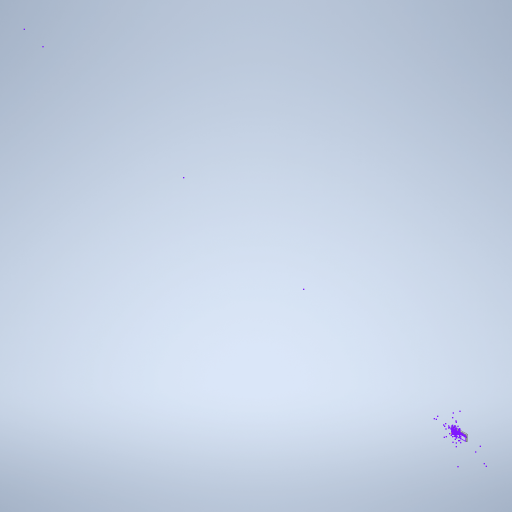
# Autodesk Inventor part: stump
Saved by Autodesk Inventor 2024 (Build 280153000, 153)
## iProperties
Created: 2023-12-16
Part Number: stump
Material: 一般
Document SubType Name: Modeling
Designer: right
Density: 1 g/cm^3
Appearance: 既定
Author: right
Autodesk Inventor part; units mm, degrees
(part 1 of 5)
ref_plane "YZ Plane" through (0, 0, 0) normal (1, 0, 0) x (0, 1, 0)
ref_plane "XZ Plane" through (0, 0, 0) normal (0, 1, 0) x (-1, 0, 0)
ref_plane "XY Plane" through (0, 0, 0) normal (0, 0, 1) x (1, 0, 0)
sketch "スケッチ1" plane through (0, 0, 0) normal (0, 0, 1) x (1, 0, 0)
  line L0 (2, 26.7042) -> (70.8408, 26.7042) construction
  line L1 (70.8408, 26.7042) -> (70.8408, 2) construction
  line L2 (70.8408, 2) -> (2, 2) construction
  line L3 (2, 2) -> (2, 26.7042) construction
  line L4 (0, 28.7042) -> (72.8408, 28.7042)
  line L5 (72.8408, 28.7042) -> (72.8408, 0)
  line L6 (72.8408, 0) -> (0, 0)
  line L7 (0, 0) -> (0, 28.7042)
  point P0 (36.4204, 28.7042)
  point P1 (0, 14.3521)
  point P2 (72.8408, 14.3521)
  dimension "d0" = 2
  dimension "d1" = 2
  dimension "d2" = 2
  dimension "d3" = 2
  dimension "d4" = 24.7042
  dimension "d5" = 68.8408
  constraints: 8 end point, 3 midpoint, 2 parallel, 1 coincident, 1 horizontal, 1 perpendicular, 2 other
  measures "d0" distance between parallel lines of L4 L0
  measures "d1" distance between parallel lines of L3 L7
  measures "d2" distance between parallel lines of L5 L1
  measures "d3" distance between parallel lines of L2 L6
  measures "d4" distance of L2.end L0.start
  measures "d5" distance of L0.start L0.end
extrude "押し出し1" add sketch "スケッチ1" along normal blind 5
sketch "スケッチ3" plane through (0, 0, 5) normal (0, 0, 1) x (1, 0, 0)
  line L0 (4.2953, 20.9134) -> (4.2763, 20.7484)
  line L1 (4.2763, 20.7484) -> (3.4513, 20.7317)
  line L2 (3.4513, 20.7317) -> (2.6263, 20.715)
  line L3 (2.6263, 20.715) -> (2.6263, 20.4784)
  line L4 (2.6263, 20.4784) -> (2.6263, 20.2418)
  line L5 (2.6263, 20.2418) -> (3.4464, 20.2251)
  arc A0 (3.8346, 20.2134) -> (3.4464, 20.2251) centre (3.0385, 0.191) ccw
  arc A1 (4.0836, 20.195) -> (3.8346, 20.2134) centre (3.6895, 16.5634) ccw
  arc A2 (4.2485, 20.1707) -> (4.0836, 20.195) centre (3.8458, 18.004) ccw
  arc A3 (4.2914, 20.1334) -> (4.2485, 20.1707) centre (4.2383, 20.1158) ccw
  arc A4 (4.2735, 20.0969) -> (4.2914, 20.1334) centre (4.2638, 20.1243) ccw
  arc A5 (4.1799, 20.0746) -> (4.2735, 20.0969) centre (4.121, 20.5302) ccw
  arc A6 (4.0094, 20.0617) -> (4.1799, 20.0746) centre (3.9733, 21.6725) ccw
  arc A7 (3.7113, 20.0584) -> (4.0094, 20.0617) centre (3.7113, 33.3375) ccw
  line L6 (3.7113, 20.0584) -> (3.1063, 20.0584)
  line L7 (3.1063, 20.0584) -> (3.1063, 19.2184)
  line L8 (3.1063, 19.2184) -> (3.1063, 18.3784)
  line L9 (3.1063, 18.3784) -> (3.4513, 18.3759)
  line L10 (3.4513, 18.3759) -> (3.7963, 18.3735)
  line L11 (3.7963, 18.3735) -> (3.5375, 18.1395)
  arc A8 (3.418, 18.0423) -> (3.5375, 18.1395) centre (2.5532, 19.2279) ccw
  arc A9 (3.2722, 17.9436) -> (3.418, 18.0423) centre (1.9502, 20.0545) ccw
  arc A10 (3.1239, 17.8579) -> (3.2722, 17.9436) centre (1.9972, 19.9794) ccw
  arc A11 (2.9975, 17.8013) -> (3.1239, 17.8579) centre (2.6369, 18.7749) ccw
  arc A12 (2.9975, 17.8013) -> (2.8882, 17.7602) centre (7.4649, 5.7405) ccw
  arc A13 (2.8882, 17.7602) -> (2.7926, 17.7231) centre (5.6156, 10.5973) ccw
  arc A14 (2.7926, 17.7231) -> (2.7116, 17.6907) centre (7.9302, 4.755) ccw
  arc A15 (2.7116, 17.6907) -> (2.6949, 17.6814) centre (2.7402, 17.6199) ccw
  arc A16 (2.6949, 17.6814) -> (2.6919, 17.6673) centre (2.7013, 17.6727) ccw
  arc A17 (2.6919, 17.6673) -> (2.7367, 17.5912) centre (5.8636, 19.479) ccw
  arc A18 (2.7367, 17.5912) -> (2.7944, 17.5007) centre (4.586, 18.7076) ccw
  arc A19 (2.7944, 17.5007) -> (2.8671, 17.3963) centre (6.3161, 19.8732) ccw
  arc A20 (2.8671, 17.3963) -> (2.9831, 17.2428) centre (6.0578, 19.6877) ccw
  arc A21 (2.9831, 17.2428) -> (3.053, 17.1803) centre (3.2002, 17.4155) ccw
  arc A22 (3.053, 17.1803) -> (3.1199, 17.1636) centre (3.1123, 17.2751) ccw
  arc A23 (3.1199, 17.1636) -> (3.208, 17.1828) centre (3.0992, 17.469) ccw
  arc A24 (3.208, 17.1828) -> (3.3895, 17.2713) centre (2.8086, 18.2332) ccw
  arc A25 (3.3895, 17.2713) -> (3.6464, 17.4363) centre (0.5309, 22.0048) ccw
  arc A26 (3.6464, 17.4363) -> (3.907, 17.6251) centre (0.4768, 22.0841) ccw
  arc A27 (3.907, 17.6251) -> (4.1113, 17.7989) centre (2.2399, 19.7922) ccw
  line L12 (4.1113, 17.7989) -> (4.3063, 17.9819)
  line L13 (4.3063, 17.9819) -> (4.3063, 17.5502)
  line L14 (4.3063, 17.5502) -> (4.3063, 17.1184)
  line L15 (4.3063, 17.1184) -> (4.6063, 17.1184)
  line L16 (4.6063, 17.1184) -> (4.9063, 17.1184)
  line L17 (4.9063, 17.1184) -> (4.9063, 17.5398)
  line L18 (4.9063, 17.5398) -> (4.9063, 17.9612)
  line L19 (4.9063, 17.9612) -> (5.1947, 17.7332)
  arc A28 (5.1947, 17.7332) -> (5.3299, 17.633) centre (6.8616, 19.842) ccw
  arc A29 (5.3299, 17.633) -> (5.4996, 17.5198) centre (8.6049, 22.3563) ccw
  arc A30 (5.4996, 17.5198) -> (5.6748, 17.4117) centre (8.642, 22.4141) ccw
  arc A31 (5.6748, 17.4117) -> (5.8276, 17.3268) centre (7.2249, 20.025) ccw
  line L20 (5.8276, 17.3268) -> (6.1722, 17.1484)
  line L21 (6.1722, 17.1484) -> (6.3476, 17.3584)
  arc A32 (6.3476, 17.3584) -> (6.4148, 17.4432) centre (4.7299, 18.7098) ccw
  arc A33 (6.4148, 17.4432) -> (6.4717, 17.5243) centre (5.2305, 18.3335) ccw
  arc A34 (6.4717, 17.5243) -> (6.5143, 17.594) centre (5.2832, 18.2992) ccw
  arc A35 (6.5143, 17.594) -> (6.5236, 17.6284) centre (6.4531, 17.6291) ccw
  arc A36 (6.5236, 17.6284) -> (6.5083, 17.6587) centre (6.4867, 17.6288) ccw
  arc A37 (6.5083, 17.6587) -> (6.4283, 17.7122) centre (5.7202, 16.5665) ccw
  arc A38 (6.4283, 17.7122) -> (6.3231, 17.7711) centre (5.6981, 16.5306) ccw
  arc A39 (6.3231, 17.7711) -> (6.1982, 17.8295) centre (5.257, 15.6552) ccw
  arc A40 (6.0567, 17.8982) -> (6.1982, 17.8295) centre (6.9163, 19.4888) ccw
  arc A41 (5.9009, 17.9884) -> (6.0567, 17.8982) centre (7.526, 20.6168) ccw
  arc A42 (5.7548, 18.0847) -> (5.9009, 17.9884) centre (7.4687, 20.5241) ccw
  arc A43 (5.6442, 18.172) -> (5.7548, 18.0847) centre (6.4837, 19.1222) ccw
  line L22 (5.6442, 18.172) -> (5.4163, 18.3734)
  line L23 (5.4163, 18.3734) -> (5.7613, 18.3759)
  line L24 (5.7613, 18.3759) -> (6.1063, 18.3784)
  line L25 (6.1063, 18.3784) -> (6.1063, 19.2184)
  line L26 (6.1063, 19.2184) -> (6.1063, 20.0584)
  line L27 (6.1063, 20.0584) -> (5.5063, 20.0584)
  arc A44 (5.1853, 20.0617) -> (5.5063, 20.0584) centre (5.5063, 35.6031) ccw
  arc A45 (5.0213, 20.0756) -> (5.1853, 20.0617) centre (5.2118, 21.3458) ccw
  arc A46 (4.935, 20.1024) -> (5.0213, 20.0756) centre (5.0654, 20.3701) ccw
  arc A47 (4.9063, 20.1484) -> (4.935, 20.1024) centre (4.9574, 20.1484) ccw
  arc A48 (4.9404, 20.196) -> (4.9063, 20.1484) centre (4.9565, 20.1484) ccw
  arc A49 (5.0563, 20.2217) -> (4.9404, 20.196) centre (5.1171, 19.6747) ccw
  arc A50 (5.2734, 20.2353) -> (5.0563, 20.2217) centre (5.3051, 17.9825) ccw
  arc A51 (5.7163, 20.2384) -> (5.2734, 20.2353) centre (5.7162, -11.2951) ccw
  line L28 (5.7163, 20.2384) -> (6.5263, 20.2384)
  line L29 (6.5263, 20.2384) -> (6.5263, 20.4784)
  line L30 (6.5263, 20.4784) -> (6.5263, 20.7184)
  line L31 (6.5263, 20.7184) -> (5.7163, 20.7184)
  line L32 (5.7163, 20.7184) -> (4.9063, 20.7184)
  line L33 (4.9063, 20.7184) -> (4.9063, 20.8984)
  arc A52 (4.9063, 20.8984) -> (4.8979, 21.0074) centre (4.1924, 20.8984) ccw
  arc A53 (4.8979, 21.0074) -> (4.8666, 21.0543) centre (4.8319, 20.9972) ccw
  arc A54 (4.8666, 21.0543) -> (4.7992, 21.0746) centre (4.7936, 20.9342) ccw
  arc A55 (4.7992, 21.0746) -> (4.6103, 21.0784) centre (4.6103, 16.3512) ccw
  arc A56 (4.6103, 21.0784) -> (4.4295, 21.0742) centre (4.6103, 17.1725) ccw
  arc A57 (4.4295, 21.0742) -> (4.3551, 21.0541) centre (4.4377, 20.8964) ccw
  arc A58 (4.3551, 21.0541) -> (4.3163, 21.0085) centre (4.3922, 20.9832) ccw
  arc A59 (4.3163, 21.0085) -> (4.2953, 20.9134) centre (4.7646, 20.8594) ccw
  arc A60 (4.2646, 19.4728) -> (4.2913, 19.5034) centre (4.2414, 19.52) ccw
  arc A61 (4.2012, 19.4492) -> (4.2646, 19.4728) centre (4.115, 19.7769) ccw
  arc A62 (4.1132, 19.4335) -> (4.2012, 19.4492) centre (4.0607, 19.983) ccw
  arc A63 (4.0063, 19.4284) -> (4.1132, 19.4335) centre (4.0063, 20.5531) ccw
  arc A64 (3.8994, 19.4335) -> (4.0063, 19.4284) centre (4.0063, 20.5531) ccw
  arc A65 (3.8114, 19.4492) -> (3.8994, 19.4335) centre (3.9518, 19.983) ccw
  arc A66 (3.7479, 19.4728) -> (3.8114, 19.4492) centre (3.8976, 19.7769) ccw
  arc A67 (3.7213, 19.5034) -> (3.7479, 19.4728) centre (3.7712, 19.52) ccw
  arc A68 (3.7302, 19.5372) -> (3.7213, 19.5034) centre (3.7516, 19.5135) ccw
  arc A69 (3.7741, 19.561) -> (3.7302, 19.5372) centre (3.8009, 19.4589) ccw
  arc A70 (3.8618, 19.5746) -> (3.7741, 19.561) centre (3.8842, 19.1424) ccw
  arc A71 (4.0063, 19.5784) -> (3.8618, 19.5746) centre (4.0063, 16.7936) ccw
  arc A72 (4.1508, 19.5746) -> (4.0063, 19.5784) centre (4.0063, 16.7936) ccw
  arc A73 (4.2385, 19.561) -> (4.1508, 19.5746) centre (4.1283, 19.1424) ccw
  arc A74 (4.2824, 19.5372) -> (4.2385, 19.561) centre (4.2116, 19.4589) ccw
  arc A75 (4.2913, 19.5034) -> (4.2824, 19.5372) centre (4.261, 19.5135) ccw
  arc A76 (5.4647, 19.4729) -> (5.4916, 19.5034) centre (5.4425, 19.5196) ccw
  arc A77 (5.3927, 19.4449) -> (5.4647, 19.4729) centre (5.2397, 19.945) ccw
  arc A78 (5.2969, 19.4226) -> (5.3927, 19.4449) centre (5.182, 20.1337) ccw
  arc A79 (5.1866, 19.4101) -> (5.2969, 19.4226) centre (5.1106, 20.5756) ccw
  arc A80 (5.0427, 19.4046) -> (5.1866, 19.4101) centre (5.012, 22.0861) ccw
  arc A81 (4.9634, 19.4146) -> (5.0427, 19.4046) centre (5.0394, 19.6984) ccw
  arc A82 (4.9222, 19.441) -> (4.9634, 19.4146) centre (4.9842, 19.4924) ccw
  arc A83 (4.9063, 19.4851) -> (4.9222, 19.441) centre (4.9754, 19.4851) ccw
  arc A84 (4.9238, 19.5297) -> (4.9063, 19.4851) centre (4.9718, 19.4851) ccw
  arc A85 (4.9703, 19.5588) -> (4.9238, 19.5297) centre (5.0013, 19.4576) ccw
  arc A86 (5.0579, 19.5743) -> (4.9703, 19.5588) centre (5.0775, 19.2085) ccw
  arc A87 (5.2113, 19.5784) -> (5.0579, 19.5743) centre (5.2113, 16.7018) ccw
  arc A88 (5.3531, 19.5746) -> (5.2113, 19.5784) centre (5.2113, 16.9114) ccw
  arc A89 (5.4395, 19.5609) -> (5.3531, 19.5746) centre (5.3307, 19.1545) ccw
  arc A90 (5.4828, 19.5371) -> (5.4395, 19.5609) centre (5.4127, 19.4608) ccw
  arc A91 (5.4916, 19.5034) -> (5.4828, 19.5371) centre (5.4611, 19.5134) ccw
  arc A92 (4.2894, 18.955) -> (4.3063, 18.9784) centre (4.2816, 18.9784) ccw
  arc A93 (4.2182, 18.936) -> (4.2894, 18.955) centre (4.103, 19.5117) ccw
  arc A94 (4.1213, 18.9227) -> (4.2182, 18.936) centre (4.061, 19.722) ccw
  arc A95 (4.0063, 18.9184) -> (4.1213, 18.9227) centre (4.0063, 20.4468) ccw
  arc A96 (3.8913, 18.9227) -> (4.0063, 18.9184) centre (4.0063, 20.4468) ccw
  arc A97 (3.7944, 18.936) -> (3.8913, 18.9227) centre (3.9516, 19.722) ccw
  arc A98 (3.7231, 18.955) -> (3.7944, 18.936) centre (3.9095, 19.5117) ccw
  arc A99 (3.7063, 18.9784) -> (3.7231, 18.955) centre (3.7309, 18.9784) ccw
  arc A100 (3.7231, 19.0018) -> (3.7063, 18.9784) centre (3.7309, 18.9784) ccw
  arc A101 (3.7944, 19.0208) -> (3.7231, 19.0018) centre (3.9095, 18.4451) ccw
  arc A102 (3.8913, 19.0341) -> (3.7944, 19.0208) centre (3.9516, 18.2348) ccw
  arc A103 (4.0063, 19.0384) -> (3.8913, 19.0341) centre (4.0063, 17.51) ccw
  arc A104 (4.1213, 19.0341) -> (4.0063, 19.0384) centre (4.0063, 17.51) ccw
  arc A105 (4.2182, 19.0208) -> (4.1213, 19.0341) centre (4.061, 18.2348) ccw
  arc A106 (4.2894, 19.0018) -> (4.2182, 19.0208) centre (4.103, 18.4451) ccw
  arc A107 (4.3063, 18.9784) -> (4.2894, 19.0018) centre (4.2816, 18.9784) ccw
  arc A108 (5.4894, 18.955) -> (5.5063, 18.9784) centre (5.4816, 18.9784) ccw
  arc A109 (5.4182, 18.936) -> (5.4894, 18.955) centre (5.303, 19.5117) ccw
  arc A110 (5.3213, 18.9227) -> (5.4182, 18.936) centre (5.261, 19.722) ccw
  arc A111 (5.2063, 18.9184) -> (5.3213, 18.9227) centre (5.2063, 20.4468) ccw
  arc A112 (5.0913, 18.9227) -> (5.2063, 18.9184) centre (5.2063, 20.4468) ccw
  arc A113 (4.9944, 18.936) -> (5.0913, 18.9227) centre (5.1516, 19.722) ccw
  arc A114 (4.9231, 18.955) -> (4.9944, 18.936) centre (5.1095, 19.5117) ccw
  arc A115 (4.9063, 18.9784) -> (4.9231, 18.955) centre (4.9309, 18.9784) ccw
  arc A116 (4.9231, 19.0018) -> (4.9063, 18.9784) centre (4.9309, 18.9784) ccw
  arc A117 (4.9944, 19.0208) -> (4.9231, 19.0018) centre (5.1095, 18.4451) ccw
  arc A118 (5.0913, 19.0341) -> (4.9944, 19.0208) centre (5.1516, 18.2348) ccw
  arc A119 (5.2063, 19.0384) -> (5.0913, 19.0341) centre (5.2063, 17.51) ccw
  arc A120 (5.3213, 19.0341) -> (5.2063, 19.0384) centre (5.2063, 17.51) ccw
  arc A121 (5.4182, 19.0208) -> (5.3213, 19.0341) centre (5.261, 18.2348) ccw
  arc A122 (5.4894, 19.0018) -> (5.4182, 19.0208) centre (5.303, 18.4451) ccw
  arc A123 (5.5063, 18.9784) -> (5.4894, 19.0018) centre (5.4816, 18.9784) ccw
  line L34 (8.6863, 20.8684) -> (8.6863, 20.6584)
  line L35 (8.6863, 20.6584) -> (7.8463, 20.6584)
  line L36 (7.8463, 20.6584) -> (7.0063, 20.6584)
  line L37 (7.0063, 20.6584) -> (7.0063, 20.3884)
  line L38 (7.0063, 20.3884) -> (7.0063, 20.1184)
  line L39 (7.0063, 20.1184) -> (8.9563, 20.1184)
  line L40 (8.9563, 20.1184) -> (10.9063, 20.1184)
  line L41 (10.9063, 20.1184) -> (10.9063, 20.3884)
  line L42 (10.9063, 20.3884) -> (10.9063, 20.6584)
  line L43 (10.9063, 20.6584) -> (10.0963, 20.6584)
  line L44 (10.0963, 20.6584) -> (9.2863, 20.6584)
  line L45 (9.2863, 20.6584) -> (9.2863, 20.8684)
  line L46 (9.2863, 20.8684) -> (9.2863, 21.0784)
  line L47 (9.2863, 21.0784) -> (8.9863, 21.0784)
  line L48 (8.9863, 21.0784) -> (8.6863, 21.0784)
  line L49 (8.6863, 21.0784) -> (8.6863, 20.8684)
  line L50 (12.1063, 20.8384) -> (12.1063, 20.5984)
  line L51 (12.1063, 20.5984) -> (11.8063, 20.5984)
  line L52 (11.8063, 20.5984) -> (11.5063, 20.5984)
  line L53 (11.5063, 20.5984) -> (11.5063, 20.3284)
  line L54 (11.5063, 20.3284) -> (11.5063, 20.0584)
  line L55 (11.5063, 20.0584) -> (11.8063, 20.0584)
  arc A124 (11.9213, 20.0541) -> (11.8063, 20.0584) centre (11.8063, 18.53) ccw
  arc A125 (12.0182, 20.0408) -> (11.9213, 20.0541) centre (11.861, 19.2548) ccw
  arc A126 (12.0894, 20.0218) -> (12.0182, 20.0408) centre (11.903, 19.4651) ccw
  arc A127 (12.1063, 19.9984) -> (12.0894, 20.0218) centre (12.0816, 19.9984) ccw
  arc A128 (12.0881, 19.9747) -> (12.1063, 19.9984) centre (12.0817, 19.9984) ccw
  arc A129 (12.0013, 19.9559) -> (12.0881, 19.9747) centre (11.8495, 20.8665) ccw
  arc A130 (11.8853, 19.9427) -> (12.0013, 19.9559) centre (11.8157, 21.0694) ccw
  arc A131 (11.7463, 19.9384) -> (11.8853, 19.9427) centre (11.7463, 22.1938) ccw
  line L56 (11.7463, 19.9384) -> (11.3863, 19.9384)
  line L57 (11.3863, 19.9384) -> (11.3863, 19.6684)
  line L58 (11.3863, 19.6684) -> (11.3863, 19.3984)
  line L59 (11.3863, 19.3984) -> (11.8167, 19.3984)
  line L60 (11.8167, 19.3984) -> (12.2472, 19.3984)
  line L61 (12.2472, 19.3984) -> (12.1159, 19.2586)
  arc A132 (12.0459, 19.1953) -> (12.1159, 19.2586) centre (11.6911, 19.6577) ccw
  arc A133 (11.9396, 19.1189) -> (12.0459, 19.1953) centre (10.7798, 20.8453) ccw
  arc A134 (11.8188, 19.0431) -> (11.9396, 19.1189) centre (10.6517, 21.0359) ccw
  arc A135 (11.7004, 18.9795) -> (11.8188, 19.0431) centre (10.8993, 20.6131) ccw
  arc A136 (11.7004, 18.9795) -> (11.5902, 18.9251) centre (22.1341, -2.2983) ccw
  arc A137 (11.5902, 18.9251) -> (11.4945, 18.8771) centre (17.6879, 6.6513) ccw
  arc A138 (11.4945, 18.8771) -> (11.4126, 18.8354) centre (25.1822, -8.1426) ccw
  arc A139 (11.4126, 18.8354) -> (11.3986, 18.8266) centre (11.4539, 18.7545) ccw
  arc A140 (11.3986, 18.8266) -> (11.3934, 18.8135) centre (11.4069, 18.8157) ccw
  arc A141 (11.3934, 18.8135) -> (11.4069, 18.7341) centre (15.6569, 19.5007) ccw
  arc A142 (11.4069, 18.7341) -> (11.426, 18.64) centre (13.6642, 19.1413) ccw
  arc A143 (11.426, 18.64) -> (11.4519, 18.5309) centre (15.5791, 19.5701) ccw
  arc A144 (11.4519, 18.5309) -> (11.4937, 18.3833) centre (13.9854, 19.1688) ccw
  arc A145 (11.4937, 18.3833) -> (11.5309, 18.3093) centre (11.7412, 18.4613) ccw
  arc A146 (11.5309, 18.3093) -> (11.5753, 18.2784) centre (11.5972, 18.3573) ccw
  arc A147 (11.5753, 18.2784) -> (11.6346, 18.278) centre (11.6058, 18.3882) ccw
  arc A148 (11.6941, 18.2678) -> (11.6346, 18.278) centre (11.6532, 18.2071) ccw
  arc A149 (11.7291, 18.2158) -> (11.6941, 18.2678) centre (11.6475, 18.1988) ccw
  arc A150 (11.7436, 18.0852) -> (11.7291, 18.2158) centre (11.0515, 18.0744) ccw
  arc A151 (11.7463, 17.7428) -> (11.7436, 18.0852) centre (-10.0958, 17.7428) ccw
  line L62 (11.7463, 17.7428) -> (11.7463, 17.1784)
  line L63 (11.7463, 17.1784) -> (12.0463, 17.1784)
  arc A152 (12.0463, 17.1784) -> (12.2148, 17.1823) centre (12.0463, 20.8261) ccw
  arc A153 (12.2148, 17.1823) -> (12.2938, 17.1994) centre (12.2036, 17.4248) ccw
  arc A154 (12.2938, 17.1994) -> (12.3322, 17.2356) centre (12.267, 17.2664) ccw
  arc A155 (12.3322, 17.2356) -> (12.3463, 17.2984) centre (12.1989, 17.2984) ccw
  arc A156 (12.3683, 17.3633) -> (12.3463, 17.2984) centre (12.4527, 17.2984) ccw
  arc A157 (12.425, 17.3999) -> (12.3683, 17.3633) centre (12.4481, 17.302) ccw
  arc A158 (12.5482, 17.4154) -> (12.425, 17.3999) centre (12.5597, 16.8274) ccw
  arc A159 (12.8563, 17.4184) -> (12.5482, 17.4154) centre (12.8563, 1.6492) ccw
  line L64 (12.8563, 17.4184) -> (13.3663, 17.4184)
  line L65 (13.3663, 17.4184) -> (13.3663, 18.2884)
  line L66 (13.3663, 18.2884) -> (13.3663, 19.1584)
  line L67 (13.3663, 19.1584) -> (13.087, 19.1584)
  arc A160 (12.9007, 19.1601) -> (13.087, 19.1584) centre (13.087, 29.2397) ccw
  arc A161 (12.8581, 19.174) -> (12.9007, 19.1601) centre (12.9021, 19.2365) ccw
  arc A162 (12.8536, 19.2022) -> (12.8581, 19.174) centre (12.8696, 19.1903) ccw
  arc A163 (12.9163, 19.2784) -> (12.8536, 19.2022) centre (13.6915, 18.5768) ccw
  arc A164 (12.9789, 19.3313) -> (12.9163, 19.2784) centre (13.1448, 19.0716) ccw
  arc A165 (13.0561, 19.3688) -> (12.9789, 19.3313) centre (13.178, 19.0196) ccw
  arc A166 (13.1494, 19.3911) -> (13.0561, 19.3688) centre (13.2117, 18.9231) ccw
  arc A167 (13.26, 19.3984) -> (13.1494, 19.3911) centre (13.26, 18.5599) ccw
  line L68 (13.26, 19.3984) -> (13.4952, 19.3984)
  line L69 (13.4952, 19.3984) -> (13.4792, 19.6989)
  arc A168 (13.478, 19.8229) -> (13.4792, 19.6989) centre (14.9277, 19.7758) ccw
  arc A169 (13.4881, 19.9345) -> (13.478, 19.8229) centre (14.446, 19.7914) ccw
  arc A170 (13.5071, 20.0236) -> (13.4881, 19.9345) centre (14.2099, 19.8267) ccw
  arc A171 (13.5348, 20.0709) -> (13.5071, 20.0236) centre (13.6112, 19.9945) ccw
  arc A172 (13.5721, 20.0577) -> (13.5348, 20.0709) centre (13.5503, 20.0554) ccw
  arc A173 (13.5913, 19.8102) -> (13.5721, 20.0577) centre (9.1456, 19.5895) ccw
  arc A174 (13.6033, 19.3928) -> (13.5913, 19.8102) centre (3.594, 19.314) ccw
  arc A175 (13.6063, 18.6304) -> (13.6033, 19.3928) centre (-83.1975, 18.6304) ccw
  line L70 (13.6063, 18.6304) -> (13.6063, 17.1184)
  line L71 (13.6063, 17.1184) -> (13.9063, 17.1184)
  line L72 (13.9063, 17.1184) -> (14.2063, 17.1184)
  line L73 (14.2063, 17.1184) -> (14.2063, 18.7084)
  line L74 (14.2063, 18.7084) -> (14.2063, 20.2984)
  line L75 (14.2063, 20.2984) -> (14.4434, 20.2984)
  line L76 (14.4434, 20.2984) -> (14.6805, 20.2984)
  line L77 (14.6805, 20.2984) -> (14.593, 20.0134)
  arc A176 (14.5546, 19.8882) -> (14.593, 20.0134) centre (-1289.7906, 420.4583) ccw
  arc A177 (14.5113, 19.7473) -> (14.5546, 19.8882) centre (-2056.7606, 655.9978) ccw
  arc A178 (14.4699, 19.6126) -> (14.5113, 19.7473) centre (-1967.312, 628.522) ccw
  arc A179 (14.4378, 19.5079) -> (14.4699, 19.6126) centre (-712.7507, 243.0535) ccw
  arc A180 (14.4378, 19.5079) -> (14.4081, 19.3727) centre (15.244, 19.26) ccw
  arc A181 (14.4081, 19.3727) -> (14.4088, 19.2573) centre (14.8181, 19.3174) ccw
  arc A182 (14.4088, 19.2573) -> (14.4428, 19.1194) centre (15.1413, 19.3649) ccw
  arc A183 (14.4428, 19.1194) -> (14.5281, 18.8922) centre (19.778, 20.9939) ccw
  arc A184 (14.6638, 18.5071) -> (14.5281, 18.8922) centre (10.0238, 17.089) ccw
  arc A185 (14.6749, 18.2941) -> (14.6638, 18.5071) centre (14.2424, 18.3783) ccw
  arc A186 (14.5827, 18.1798) -> (14.6749, 18.2941) centre (14.5207, 18.3241) ccw
  arc A187 (14.3814, 18.1384) -> (14.5827, 18.1798) centre (14.3814, 18.6487) ccw
  arc A188 (14.3814, 18.1384) -> (14.3039, 18.126) centre (14.3814, 17.8911) ccw
  arc A189 (14.3039, 18.126) -> (14.2749, 18.0893) centre (14.3173, 18.0856) ccw
  arc A190 (14.2749, 18.0893) -> (14.2823, 18.0105) centre (14.4947, 18.0701) ccw
  arc A191 (14.2823, 18.0105) -> (14.35, 17.7784) centre (25.3033, 21.1009) ccw
  arc A192 (14.35, 17.7784) -> (14.4059, 17.613) centre (17.0017, 18.5827) ccw
  arc A193 (14.4059, 17.613) -> (14.4515, 17.5474) centre (14.5573, 17.6696) ccw
  arc A194 (14.4515, 17.5474) -> (14.5184, 17.5192) centre (14.5283, 17.6361) ccw
  arc A195 (14.5184, 17.5192) -> (14.6535, 17.5156) centre (14.616, 18.6659) ccw
  arc A196 (14.6535, 17.5156) -> (14.9602, 17.5767) centre (14.6223, 18.4729) ccw
  arc A197 (14.9602, 17.5767) -> (15.1627, 17.7314) centre (14.8039, 17.9913) ccw
  arc A198 (15.1627, 17.7314) -> (15.265, 17.9912) centre (14.7089, 18.0601) ccw
  arc A199 (15.265, 17.9912) -> (15.2712, 18.3686) centre (13.5086, 18.2088) ccw
  arc A200 (15.2712, 18.3686) -> (15.2496, 18.5236) centre (13.652, 18.2218) ccw
  arc A201 (15.2496, 18.5236) -> (15.21, 18.7037) centre (12.1768, 17.9432) ccw
  arc A202 (15.21, 18.7037) -> (15.1602, 18.8801) centre (12.2004, 17.9491) ccw
  arc A203 (15.1602, 18.8801) -> (15.107, 19.0234) centre (13.7239, 18.4283) ccw
  line L78 (15.107, 19.0234) -> (14.9743, 19.332)
  line L79 (14.9743, 19.332) -> (15.167, 19.9104)
  line L80 (15.167, 19.9104) -> (15.3597, 20.4889)
  line L81 (15.3597, 20.4889) -> (15.1612, 20.6936)
  line L82 (15.1612, 20.6936) -> (14.9627, 20.8984)
  line L83 (14.9627, 20.8984) -> (14.2845, 20.8984)
  line L84 (14.2845, 20.8984) -> (13.6063, 20.8984)
  line L85 (13.6063, 20.8984) -> (13.6063, 20.7484)
  arc A204 (13.5986, 20.6416) -> (13.6063, 20.7484) centre (12.8634, 20.7484) ccw
  arc A205 (13.5679, 20.6062) -> (13.5986, 20.6416) centre (13.5557, 20.6478) ccw
  arc A206 (13.5164, 20.6153) -> (13.5679, 20.6062) centre (13.5513, 20.6627) ccw
  arc A207 (13.4203, 20.6938) -> (13.5164, 20.6153) centre (14.2406, 21.6002) ccw
  arc A208 (13.4203, 20.6938) -> (13.3559, 20.7423) centre (13.1202, 20.3621) ccw
  arc A209 (13.3559, 20.7423) -> (13.3148, 20.7442) centre (13.3336, 20.7063) ccw
  arc A210 (13.3148, 20.7442) -> (13.2758, 20.7081) centre (13.3566, 20.66) ccw
  arc A211 (13.2758, 20.7081) -> (13.2086, 20.5888) centre (15.6357, 19.3012) ccw
  arc A212 (13.1538, 20.4911) -> (13.2086, 20.5888) centre (11.1034, 21.7056) ccw
  arc A213 (13.1203, 20.454) -> (13.1538, 20.4911) centre (13.0451, 20.5555) ccw
  arc A214 (13.097, 20.457) -> (13.1203, 20.454) centre (13.1103, 20.4675) ccw
  arc A215 (13.0799, 20.4934) -> (13.097, 20.457) centre (13.166, 20.5118) ccw
  arc A216 (13.0799, 20.4934) -> (13.0587, 20.5395) centre (12.9667, 20.4692) ccw
  arc A217 (13.0587, 20.5395) -> (13.0197, 20.5725) centre (12.9638, 20.467) ccw
  arc A218 (13.0197, 20.5725) -> (12.9611, 20.5921) centre (12.9315, 20.4061) ccw
  arc A219 (12.9611, 20.5921) -> (12.8819, 20.5984) centre (12.8819, 20.0954) ccw
  arc A220 (12.7788, 20.6059) -> (12.8819, 20.5984) centre (12.8819, 21.3128) ccw
  arc A221 (12.7323, 20.6339) -> (12.7788, 20.6059) centre (12.7889, 20.6754) ccw
  arc A222 (12.7109, 20.693) -> (12.7323, 20.6339) centre (12.8226, 20.7) ccw
  arc A223 (12.7063, 20.8384) -> (12.7109, 20.693) centre (15.0138, 20.8384) ccw
  line L86 (12.7063, 20.8384) -> (12.7063, 21.0784)
  line L87 (12.7063, 21.0784) -> (12.4063, 21.0784)
  line L88 (12.4063, 21.0784) -> (12.1063, 21.0784)
  line L89 (12.1063, 21.0784) -> (12.1063, 20.8384)
  arc A224 (12.8217, 19.9755) -> (12.8263, 19.9984) centre (12.7668, 19.9984) ccw
  arc A225 (12.8087, 19.956) -> (12.8217, 19.9755) centre (12.7659, 19.9987) ccw
  arc A226 (12.7892, 19.943) -> (12.8087, 19.956) centre (12.7659, 19.9987) ccw
  arc A227 (12.7663, 19.9384) -> (12.7892, 19.943) centre (12.7663, 19.9979) ccw
  arc A228 (12.7434, 19.943) -> (12.7663, 19.9384) centre (12.7663, 19.9979) ccw
  arc A229 (12.7239, 19.956) -> (12.7434, 19.943) centre (12.7666, 19.9987) ccw
  arc A230 (12.7109, 19.9755) -> (12.7239, 19.956) centre (12.7666, 19.9987) ccw
  arc A231 (12.7063, 19.9984) -> (12.7109, 19.9755) centre (12.7658, 19.9984) ccw
  arc A232 (12.7109, 20.0213) -> (12.7063, 19.9984) centre (12.7658, 19.9984) ccw
  arc A233 (12.7239, 20.0408) -> (12.7109, 20.0213) centre (12.7666, 19.9981) ccw
  arc A234 (12.7434, 20.0538) -> (12.7239, 20.0408) centre (12.7666, 19.9981) ccw
  arc A235 (12.7663, 20.0584) -> (12.7434, 20.0538) centre (12.7663, 19.9989) ccw
  arc A236 (12.7892, 20.0538) -> (12.7663, 20.0584) centre (12.7663, 19.9989) ccw
  arc A237 (12.8087, 20.0408) -> (12.7892, 20.0538) centre (12.7659, 19.9981) ccw
  arc A238 (12.8217, 20.0213) -> (12.8087, 20.0408) centre (12.7659, 19.9981) ccw
  arc A239 (12.8263, 19.9984) -> (12.8217, 20.0213) centre (12.7668, 19.9984) ccw
  arc A240 (12.7556, 18.5582) -> (12.7663, 18.6184) centre (12.5909, 18.6184) ccw
  arc A241 (12.725, 18.522) -> (12.7556, 18.5582) centre (12.6908, 18.5819) ccw
  arc A242 (12.6657, 18.5033) -> (12.725, 18.522) centre (12.6526, 18.6487) ccw
  arc A243 (12.5563, 18.4984) -> (12.6657, 18.5033) centre (12.5563, 19.7157) ccw
  arc A244 (12.4468, 18.5033) -> (12.5563, 18.4984) centre (12.5563, 19.7157) ccw
  arc A245 (12.3875, 18.522) -> (12.4468, 18.5033) centre (12.4599, 18.6487) ccw
  arc A246 (12.3569, 18.5582) -> (12.3875, 18.522) centre (12.4218, 18.5819) ccw
  arc A247 (12.3463, 18.6184) -> (12.3569, 18.5582) centre (12.5216, 18.6184) ccw
  arc A248 (12.3569, 18.6785) -> (12.3463, 18.6184) centre (12.5216, 18.6184) ccw
  arc A249 (12.3875, 18.7148) -> (12.3569, 18.6785) centre (12.4218, 18.6549) ccw
  arc A250 (12.4468, 18.7335) -> (12.3875, 18.7148) centre (12.4599, 18.5881) ccw
  arc A251 (12.5563, 18.7384) -> (12.4468, 18.7335) centre (12.5563, 17.5211) ccw
  arc A252 (12.6657, 18.7335) -> (12.5563, 18.7384) centre (12.5563, 17.5211) ccw
  arc A253 (12.725, 18.7148) -> (12.6657, 18.7335) centre (12.6526, 18.5881) ccw
  arc A254 (12.7556, 18.6785) -> (12.725, 18.7148) centre (12.6908, 18.6549) ccw
  arc A255 (12.7663, 18.6184) -> (12.7556, 18.6785) centre (12.5909, 18.6184) ccw
  arc A256 (12.7556, 17.8982) -> (12.7663, 17.9584) centre (12.5909, 17.9584) ccw
  arc A257 (12.725, 17.862) -> (12.7556, 17.8982) centre (12.6908, 17.9219) ccw
  arc A258 (12.6657, 17.8433) -> (12.725, 17.862) centre (12.6526, 17.9887) ccw
  arc A259 (12.5563, 17.8384) -> (12.6657, 17.8433) centre (12.5563, 19.0557) ccw
  arc A260 (12.4468, 17.8433) -> (12.5563, 17.8384) centre (12.5563, 19.0557) ccw
  arc A261 (12.3875, 17.862) -> (12.4468, 17.8433) centre (12.4599, 17.9887) ccw
  arc A262 (12.3569, 17.8982) -> (12.3875, 17.862) centre (12.4218, 17.9219) ccw
  arc A263 (12.3463, 17.9584) -> (12.3569, 17.8982) centre (12.5216, 17.9584) ccw
  arc A264 (12.3569, 18.0185) -> (12.3463, 17.9584) centre (12.5216, 17.9584) ccw
  arc A265 (12.3875, 18.0548) -> (12.3569, 18.0185) centre (12.4218, 17.9949) ccw
  arc A266 (12.4468, 18.0735) -> (12.3875, 18.0548) centre (12.4599, 17.9281) ccw
  arc A267 (12.5563, 18.0784) -> (12.4468, 18.0735) centre (12.5563, 16.8611) ccw
  arc A268 (12.6657, 18.0735) -> (12.5563, 18.0784) centre (12.5563, 16.8611) ccw
  arc A269 (12.725, 18.0548) -> (12.6657, 18.0735) centre (12.6526, 17.9281) ccw
  arc A270 (12.7556, 18.0185) -> (12.725, 18.0548) centre (12.6908, 17.9949) ccw
  arc A271 (12.7663, 17.9584) -> (12.7556, 18.0185) centre (12.5909, 17.9584) ccw
  arc A272 (15.9787, 20.8213) -> (15.9036, 20.7098) centre (17.7557, 19.544) ccw
  arc A273 (15.9036, 20.7098) -> (15.8642, 20.6304) centre (16.2753, 20.4758) ccw
  arc A274 (15.8642, 20.6304) -> (15.8564, 20.5786) centre (15.9824, 20.586) ccw
  arc A275 (15.8564, 20.5786) -> (15.8772, 20.5514) centre (15.8869, 20.5804) ccw
  arc A276 (15.9217, 20.5314) -> (15.8772, 20.5514) centre (15.8005, 20.3213) ccw
  arc A277 (16.019, 20.4739) -> (15.9217, 20.5314) centre (13.3162, 16.013) ccw
  arc A278 (16.1335, 20.4024) -> (16.019, 20.4739) centre (13.3762, 16.1121) ccw
  arc A279 (16.2551, 20.3225) -> (16.1335, 20.4024) centre (12.4103, 14.6091) ccw
  arc A280 (16.2551, 20.3225) -> (16.3725, 20.2442) centre (24.8724, 33.1278) ccw
  arc A281 (16.3725, 20.2442) -> (16.474, 20.1783) centre (20.9882, 27.2404) ccw
  arc A282 (16.474, 20.1783) -> (16.5629, 20.1217) centre (31.7094, 44.0124) ccw
  arc A283 (16.5629, 20.1217) -> (16.5743, 20.1184) centre (16.5743, 20.1397) ccw
  arc A284 (16.5743, 20.1184) -> (16.584, 20.1233) centre (16.5743, 20.1305) ccw
  arc A285 (16.584, 20.1233) -> (16.6309, 20.1869) centre (9.9601, 25.0593) ccw
  arc A286 (16.6309, 20.1869) -> (16.6843, 20.2621) centre (14.0059, 22.1042) ccw
  arc A287 (16.6843, 20.2621) -> (16.7446, 20.3515) centre (11.7135, 23.6809) ccw
  line L90 (16.7446, 20.3515) -> (16.8988, 20.5845)
  line L91 (16.8988, 20.5845) -> (16.7675, 20.7047)
  arc A288 (16.7675, 20.7047) -> (16.7004, 20.7592) centre (16.2704, 20.1617) ccw
  arc A289 (16.7004, 20.7592) -> (16.6041, 20.825) centre (15.3138, 18.8325) ccw
  arc A290 (16.6041, 20.825) -> (16.4973, 20.8906) centre (15.1973, 18.6524) ccw
  arc A291 (16.4973, 20.8906) -> (16.3955, 20.9456) centre (15.5514, 19.262) ccw
  line L92 (16.3955, 20.9456) -> (16.1548, 21.0663)
  line L93 (16.1548, 21.0663) -> (15.9787, 20.8213)
  line L94 (27.4663, 19.0984) -> (27.4663, 17.1184)
  line L95 (27.4663, 17.1184) -> (27.7663, 17.1184)
  line L96 (27.7663, 17.1184) -> (28.0663, 17.1184)
  line L97 (28.0663, 17.1184) -> (28.0663, 19.0984)
  line L98 (28.0663, 19.0984) -> (28.0663, 21.0784)
  line L99 (28.0663, 21.0784) -> (27.7663, 21.0784)
  line L100 (27.7663, 21.0784) -> (27.4663, 21.0784)
  line L101 (27.4663, 21.0784) -> (27.4663, 19.0984)
  line L102 (34.8463, 20.8984) -> (34.8463, 20.7184)
  line L103 (34.8463, 20.7184) -> (34.0063, 20.7184)
  line L104 (34.0063, 20.7184) -> (33.1663, 20.7184)
  line L105 (33.1663, 20.7184) -> (33.1663, 20.4784)
  line L106 (33.1663, 20.4784) -> (33.1663, 20.2384)
  line L107 (33.1663, 20.2384) -> (34.0063, 20.2384)
  arc A292 (34.4665, 20.2353) -> (34.0063, 20.2384) centre (34.0063, -14.0591) ccw
  arc A293 (34.6913, 20.2218) -> (34.4665, 20.2353) centre (34.4341, 17.8219) ccw
  arc A294 (34.8115, 20.1962) -> (34.6913, 20.2218) centre (34.6277, 19.6282) ccw
  arc A295 (34.8463, 20.1484) -> (34.8115, 20.1962) centre (34.7961, 20.1484) ccw
  arc A296 (34.8185, 20.1027) -> (34.8463, 20.1484) centre (34.7949, 20.1484) ccw
  arc A297 (34.7363, 20.0758) -> (34.8185, 20.1027) centre (34.694, 20.3435) ccw
  arc A298 (34.5799, 20.0618) -> (34.7363, 20.0758) centre (34.5541, 21.2298) ccw
  arc A299 (34.2763, 20.0584) -> (34.5799, 20.0618) centre (34.2763, 33.7904) ccw
  line L108 (34.2763, 20.0584) -> (33.7063, 20.0584)
  line L109 (33.7063, 20.0584) -> (33.7063, 19.2184)
  line L110 (33.7063, 19.2184) -> (33.7063, 18.3784)
  line L111 (33.7063, 18.3784) -> (34.0513, 18.376)
  line L112 (34.0513, 18.376) -> (34.3963, 18.3735)
  line L113 (34.3963, 18.3735) -> (34.1863, 18.1892)
  arc A300 (34.0795, 18.106) -> (34.1863, 18.1892) centre (33.4136, 19.0698) ccw
  arc A301 (33.9277, 18.0065) -> (34.0795, 18.106) centre (31.976, 21.1504) ccw
  arc A302 (33.76, 17.9079) -> (33.9277, 18.0065) centre (31.8057, 21.4248) ccw
  arc A303 (33.6009, 17.8258) -> (33.76, 17.9079) centre (32.3567, 20.4333) ccw
  line L114 (33.6009, 17.8258) -> (33.2255, 17.6467)
  line L115 (33.2255, 17.6467) -> (33.4174, 17.3975)
  arc A304 (33.4921, 17.3006) -> (33.4174, 17.3975) centre (-24.9743, -27.5962) ccw
  arc A305 (33.5573, 17.2154) -> (33.4921, 17.3006) centre (-1.0792, -9.247) ccw
  arc A306 (33.6129, 17.1426) -> (33.5573, 17.2154) centre (-34.9075, -35.0921) ccw
  arc A307 (33.6238, 17.1274) -> (33.6129, 17.1426) centre (33.3158, 16.9161) ccw
  arc A308 (33.6238, 17.1274) -> (33.6819, 17.1146) centre (33.6598, 17.1521) ccw
  arc A309 (33.6819, 17.1146) -> (34.0044, 17.3103) centre (25.6381, 30.7282) ccw
  arc A310 (34.0044, 17.3103) -> (34.321, 17.5209) centre (30.5663, 22.8242) ccw
  arc A311 (34.321, 17.5209) -> (34.5564, 17.709) centre (32.8213, 19.6392) ccw
  line L116 (34.5564, 17.709) -> (34.8463, 17.9695)
  line L117 (34.8463, 17.9695) -> (34.8463, 17.544)
  line L118 (34.8463, 17.544) -> (34.8463, 17.1184)
  line L119 (34.8463, 17.1184) -> (35.1463, 17.1184)
  line L120 (35.1463, 17.1184) -> (35.4463, 17.1184)
  line L121 (35.4463, 17.1184) -> (35.4463, 17.5403)
  line L122 (35.4463, 17.5403) -> (35.4463, 17.9623)
  line L123 (35.4463, 17.9623) -> (35.7613, 17.7257)
  arc A312 (35.7613, 17.7257) -> (36.0295, 17.539) centre (38.4684, 21.3293) ccw
  arc A313 (36.0295, 17.539) -> (36.3307, 17.3573) centre (39.2998, 22.6215) ccw
  arc A314 (36.3307, 17.3573) -> (36.6103, 17.2073) centre (40.0651, 23.9782) ccw
  arc A315 (36.6103, 17.2073) -> (36.7302, 17.1791) centre (36.7273, 17.4367) ccw
  arc A316 (36.7302, 17.1791) -> (36.7946, 17.2102) centre (36.7293, 17.2633) ccw
  arc A317 (36.7946, 17.2102) -> (36.9233, 17.3786) centre (33.9868, 19.49) ccw
  arc A318 (36.9233, 17.3786) -> (37.0399, 17.5535) centre (34.5099, 19.1139) ccw
  arc A319 (37.0399, 17.5535) -> (37.0663, 17.6465) centre (36.8891, 17.6465) ccw
  arc A320 (37.0663, 17.6465) -> (37.0524, 17.6719) centre (37.036, 17.6465) ccw
  arc A321 (37.0524, 17.6719) -> (36.9712, 17.7211) centre (36.1182, 16.2203) ccw
  arc A322 (36.9712, 17.7211) -> (36.8667, 17.7754) centre (36.1928, 16.3515) ccw
  arc A323 (36.8667, 17.7754) -> (36.7427, 17.8304) centre (35.6859, 15.2806) ccw
  arc A324 (36.602, 17.8966) -> (36.7427, 17.8304) centre (37.3803, 19.3688) ccw
  arc A325 (36.4462, 17.9852) -> (36.602, 17.8966) centre (37.9669, 20.478) ccw
  arc A326 (36.2996, 18.081) -> (36.4462, 17.9852) centre (37.9227, 20.4057) ccw
  arc A327 (36.1877, 18.169) -> (36.2996, 18.081) centre (37.0148, 19.1054) ccw
  line L124 (36.1877, 18.169) -> (35.9563, 18.3734)
  line L125 (35.9563, 18.3734) -> (36.3013, 18.3759)
  line L126 (36.3013, 18.3759) -> (36.6463, 18.3784)
  line L127 (36.6463, 18.3784) -> (36.6463, 19.2184)
  line L128 (36.6463, 19.2184) -> (36.6463, 20.0584)
  line L129 (36.6463, 20.0584) -> (36.0413, 20.0584)
  arc A328 (35.7431, 20.0617) -> (36.0413, 20.0584) centre (36.0413, 33.3375) ccw
  arc A329 (35.5727, 20.0746) -> (35.7431, 20.0617) centre (35.7793, 21.6725) ccw
  arc A330 (35.4791, 20.0969) -> (35.5727, 20.0746) centre (35.6316, 20.5302) ccw
  arc A331 (35.4612, 20.1334) -> (35.4791, 20.0969) centre (35.4887, 20.1243) ccw
  arc A332 (35.504, 20.1707) -> (35.4612, 20.1334) centre (35.5143, 20.1158) ccw
  arc A333 (35.669, 20.195) -> (35.504, 20.1707) centre (35.9067, 18.004) ccw
  arc A334 (35.918, 20.2134) -> (35.669, 20.195) centre (36.0631, 16.5634) ccw
  arc A335 (36.3062, 20.2251) -> (35.918, 20.2134) centre (36.714, 0.191) ccw
  line L130 (36.3062, 20.2251) -> (37.1263, 20.2418)
  line L131 (37.1263, 20.2418) -> (37.1263, 20.4784)
  line L132 (37.1263, 20.4784) -> (37.1263, 20.715)
  line L133 (37.1263, 20.715) -> (36.3013, 20.7317)
  line L134 (36.3013, 20.7317) -> (35.4763, 20.7484)
  line L135 (35.4763, 20.7484) -> (35.4573, 20.9134)
  arc A336 (35.4573, 20.9134) -> (35.4363, 21.0085) centre (34.988, 20.8594) ccw
  arc A337 (35.4363, 21.0085) -> (35.3975, 21.0541) centre (35.3604, 20.9832) ccw
  arc A338 (35.3975, 21.0541) -> (35.3231, 21.0742) centre (35.3149, 20.8964) ccw
  arc A339 (35.3231, 21.0742) -> (35.1423, 21.0784) centre (35.1423, 17.1725) ccw
  arc A340 (35.1423, 21.0784) -> (34.9533, 21.0746) centre (35.1423, 16.3512) ccw
  arc A341 (34.9533, 21.0746) -> (34.8859, 21.0543) centre (34.959, 20.9342) ccw
  arc A342 (34.8859, 21.0543) -> (34.8547, 21.0074) centre (34.9206, 20.9972) ccw
  arc A343 (34.8547, 21.0074) -> (34.8463, 20.8984) centre (35.5601, 20.8984) ccw
  arc A344 (34.8299, 19.4466) -> (34.8463, 19.4884) centre (34.7846, 19.4884) ccw
  arc A345 (34.7863, 19.4184) -> (34.8299, 19.4466) centre (34.7533, 19.5174) ccw
  arc A346 (34.7067, 19.4027) -> (34.7863, 19.4184) centre (34.6855, 19.7208) ccw
  arc A347 (34.5763, 19.3984) -> (34.7067, 19.4027) centre (34.5763, 21.3563) ccw
  arc A348 (34.4458, 19.4027) -> (34.5763, 19.3984) centre (34.5763, 21.3563) ccw
  arc A349 (34.3663, 19.4184) -> (34.4458, 19.4027) centre (34.4671, 19.7208) ccw
  arc A350 (34.3226, 19.4466) -> (34.3663, 19.4184) centre (34.3993, 19.5174) ccw
  arc A351 (34.3063, 19.4884) -> (34.3226, 19.4466) centre (34.3679, 19.4884) ccw
  arc A352 (34.3226, 19.5302) -> (34.3063, 19.4884) centre (34.3679, 19.4884) ccw
  arc A353 (34.3663, 19.5584) -> (34.3226, 19.5302) centre (34.3993, 19.4594) ccw
  arc A354 (34.4458, 19.574) -> (34.3663, 19.5584) centre (34.4671, 19.256) ccw
  arc A355 (34.5763, 19.5784) -> (34.4458, 19.574) centre (34.5763, 17.6205) ccw
  arc A356 (34.7067, 19.574) -> (34.5763, 19.5784) centre (34.5763, 17.6205) ccw
  arc A357 (34.7863, 19.5584) -> (34.7067, 19.574) centre (34.6855, 19.256) ccw
  arc A358 (34.8299, 19.5302) -> (34.7863, 19.5584) centre (34.7533, 19.4594) ccw
  arc A359 (34.8463, 19.4884) -> (34.8299, 19.5302) centre (34.7846, 19.4884) ccw
  arc A360 (36.0046, 19.4728) -> (36.0313, 19.5034) centre (35.9814, 19.52) ccw
  arc A361 (35.9412, 19.4492) -> (36.0046, 19.4728) centre (35.855, 19.7769) ccw
  arc A362 (35.8532, 19.4335) -> (35.9412, 19.4492) centre (35.8007, 19.983) ccw
  arc A363 (35.7463, 19.4284) -> (35.8532, 19.4335) centre (35.7463, 20.5531) ccw
  arc A364 (35.6394, 19.4335) -> (35.7463, 19.4284) centre (35.7463, 20.5531) ccw
  arc A365 (35.5514, 19.4492) -> (35.6394, 19.4335) centre (35.6918, 19.983) ccw
  arc A366 (35.4879, 19.4728) -> (35.5514, 19.4492) centre (35.6376, 19.7769) ccw
  arc A367 (35.4613, 19.5034) -> (35.4879, 19.4728) centre (35.5112, 19.52) ccw
  arc A368 (35.4702, 19.5372) -> (35.4613, 19.5034) centre (35.4916, 19.5135) ccw
  arc A369 (35.5141, 19.561) -> (35.4702, 19.5372) centre (35.5409, 19.4589) ccw
  arc A370 (35.6018, 19.5746) -> (35.5141, 19.561) centre (35.6242, 19.1424) ccw
  arc A371 (35.7463, 19.5784) -> (35.6018, 19.5746) centre (35.7463, 16.7936) ccw
  arc A372 (35.8908, 19.5746) -> (35.7463, 19.5784) centre (35.7463, 16.7936) ccw
  arc A373 (35.9785, 19.561) -> (35.8908, 19.5746) centre (35.8683, 19.1424) ccw
  arc A374 (36.0224, 19.5372) -> (35.9785, 19.561) centre (35.9516, 19.4589) ccw
  arc A375 (36.0313, 19.5034) -> (36.0224, 19.5372) centre (36.001, 19.5135) ccw
  arc A376 (34.8303, 18.9551) -> (34.8463, 18.9784) centre (34.8213, 18.9784) ccw
  arc A377 (34.767, 18.936) -> (34.8303, 18.9551) centre (34.6699, 19.373) ccw
  arc A378 (34.6798, 18.9227) -> (34.767, 18.936) centre (34.625, 19.5748) ccw
  arc A379 (34.5763, 18.9184) -> (34.6798, 18.9227) centre (34.5763, 20.1552) ccw
  arc A380 (34.4728, 18.9227) -> (34.5763, 18.9184) centre (34.5763, 20.1552) ccw
  arc A381 (34.3856, 18.936) -> (34.4728, 18.9227) centre (34.5275, 19.5748) ccw
  arc A382 (34.3223, 18.9551) -> (34.3856, 18.936) centre (34.4827, 19.373) ccw
  arc A383 (34.3063, 18.9784) -> (34.3223, 18.9551) centre (34.3312, 18.9784) ccw
  arc A384 (34.3223, 19.0017) -> (34.3063, 18.9784) centre (34.3312, 18.9784) ccw
  arc A385 (34.3856, 19.0208) -> (34.3223, 19.0017) centre (34.4827, 18.5838) ccw
  arc A386 (34.4728, 19.0341) -> (34.3856, 19.0208) centre (34.5275, 18.382) ccw
  arc A387 (34.5763, 19.0384) -> (34.4728, 19.0341) centre (34.5763, 17.8016) ccw
  arc A388 (34.6798, 19.0341) -> (34.5763, 19.0384) centre (34.5763, 17.8016) ccw
  arc A389 (34.767, 19.0208) -> (34.6798, 19.0341) centre (34.625, 18.382) ccw
  arc A390 (34.8303, 19.0017) -> (34.767, 19.0208) centre (34.6699, 18.5838) ccw
  arc A391 (34.8463, 18.9784) -> (34.8303, 19.0017) centre (34.8213, 18.9784) ccw
  arc A392 (36.0294, 18.955) -> (36.0463, 18.9784) centre (36.0216, 18.9784) ccw
  arc A393 (35.9582, 18.936) -> (36.0294, 18.955) centre (35.843, 19.5117) ccw
  arc A394 (35.8613, 18.9227) -> (35.9582, 18.936) centre (35.801, 19.722) ccw
  arc A395 (35.7463, 18.9184) -> (35.8613, 18.9227) centre (35.7463, 20.4468) ccw
  arc A396 (35.6313, 18.9227) -> (35.7463, 18.9184) centre (35.7463, 20.4468) ccw
  arc A397 (35.5344, 18.936) -> (35.6313, 18.9227) centre (35.6916, 19.722) ccw
  arc A398 (35.4631, 18.955) -> (35.5344, 18.936) centre (35.6495, 19.5117) ccw
  arc A399 (35.4463, 18.9784) -> (35.4631, 18.955) centre (35.4709, 18.9784) ccw
  arc A400 (35.4631, 19.0018) -> (35.4463, 18.9784) centre (35.4709, 18.9784) ccw
  arc A401 (35.5344, 19.0208) -> (35.4631, 19.0018) centre (35.6495, 18.4451) ccw
  arc A402 (35.6313, 19.0341) -> (35.5344, 19.0208) centre (35.6916, 18.2348) ccw
  arc A403 (35.7463, 19.0384) -> (35.6313, 19.0341) centre (35.7463, 17.51) ccw
  arc A404 (35.8613, 19.0341) -> (35.7463, 19.0384) centre (35.7463, 17.51) ccw
  arc A405 (35.9582, 19.0208) -> (35.8613, 19.0341) centre (35.801, 18.2348) ccw
  arc A406 (36.0294, 19.0018) -> (35.9582, 19.0208) centre (35.843, 18.4451) ccw
  arc A407 (36.0463, 18.9784) -> (36.0294, 19.0018) centre (36.0216, 18.9784) ccw
  arc A408 (38.5442, 20.8935) -> (38.5663, 20.9584) centre (38.4598, 20.9584) ccw
  arc A409 (38.4875, 20.8569) -> (38.5442, 20.8935) centre (38.4645, 20.9548) ccw
  arc A410 (38.3643, 20.8414) -> (38.4875, 20.8569) centre (38.3528, 21.4294) ccw
  arc A411 (38.0563, 20.8384) -> (38.3643, 20.8414) centre (38.0563, 36.6076) ccw
  line L136 (38.0563, 20.8384) -> (37.5463, 20.8384)
  line L137 (37.5463, 20.8384) -> (37.5463, 20.5984)
  line L138 (37.5463, 20.5984) -> (37.5463, 20.3584)
  line L139 (37.5463, 20.3584) -> (38.0227, 20.3584)
  arc A412 (38.208, 20.354) -> (38.0227, 20.3584) centre (38.0227, 16.4163) ccw
  arc A413 (38.3701, 20.3408) -> (38.208, 20.354) centre (38.0976, 18.0085) ccw
  arc A414 (38.501, 20.3221) -> (38.3701, 20.3408) centre (38.0677, 17.7522) ccw
  arc A415 (38.5363, 20.2984) -> (38.501, 20.3221) centre (38.4925, 20.2713) ccw
  arc A416 (38.5325, 20.2742) -> (38.5363, 20.2984) centre (38.5203, 20.2885) ccw
  arc A417 (38.4966, 20.2548) -> (38.5325, 20.2742) centre (38.4696, 20.3476) ccw
  arc A418 (38.4276, 20.2422) -> (38.4966, 20.2548) centre (38.4008, 20.5844) ccw
  arc A419 (38.3298, 20.2384) -> (38.4276, 20.2422) centre (38.3298, 21.4914) ccw
  line L140 (38.3298, 20.2384) -> (38.0863, 20.2384)
  line L141 (38.0863, 20.2384) -> (38.0863, 19.6084)
  arc A420 (38.0863, 19.6084) -> (38.0891, 19.2204) centre (65.0705, 19.6084) ccw
  arc A421 (38.0891, 19.2204) -> (38.1041, 19.0721) centre (38.9471, 19.2327) ccw
  arc A422 (38.1041, 19.0721) -> (38.1407, 19.0048) centre (38.228, 19.0957) ccw
  arc A423 (38.1407, 19.0048) -> (38.2063, 18.9784) centre (38.2063, 19.0731) ccw
  arc A424 (38.2522, 18.9739) -> (38.2063, 18.9784) centre (38.2063, 18.743) ccw
  arc A425 (38.291, 18.9604) -> (38.2522, 18.9739) centre (38.2231, 18.8274) ccw
  arc A426 (38.3172, 18.9405) -> (38.291, 18.9604) centre (38.2488, 18.8778) ccw
  arc A427 (38.3263, 18.9171) -> (38.3172, 18.9405) centre (38.2916, 18.9171) ccw
  arc A428 (38.2899, 18.8464) -> (38.3263, 18.9171) centre (38.2394, 18.9171) ccw
  arc A429 (38.0482, 18.6808) -> (38.2899, 18.8464) centre (34.0483, 24.7781) ccw
  arc A430 (37.8037, 18.5296) -> (38.0482, 18.6808) centre (35.104, 23.1688) ccw
  arc A431 (37.6881, 18.4984) -> (37.8037, 18.5296) centre (37.6881, 18.7283) ccw
  arc A432 (37.6881, 18.4984) -> (37.6118, 18.4729) centre (37.6881, 18.3717) ccw
  arc A433 (37.6118, 18.4729) -> (37.5781, 18.4098) centre (37.663, 18.405) ccw
  arc A434 (37.5781, 18.4098) -> (37.595, 18.2998) centre (37.8455, 18.3946) ccw
  arc A435 (37.595, 18.2998) -> (37.6676, 18.1359) centre (39.1201, 18.8769) ccw
  arc A436 (37.6676, 18.1359) -> (37.7517, 17.9785) centre (41.7838, 20.2358) ccw
  arc A437 (37.7517, 17.9785) -> (37.7961, 17.9344) centre (37.8514, 18.0344) ccw
  arc A438 (37.7961, 17.9344) -> (37.8465, 17.9328) centre (37.8228, 17.9826) ccw
  arc A439 (37.8465, 17.9328) -> (37.9398, 17.9852) centre (37.5103, 18.6407) ccw
  line L142 (37.9398, 17.9852) -> (38.0863, 18.0812)
  line L143 (38.0863, 18.0812) -> (38.0863, 17.6298)
  line L144 (38.0863, 17.6298) -> (38.0863, 17.1784)
  line L145 (38.0863, 17.1784) -> (38.3863, 17.1784)
  arc A440 (38.3863, 17.1784) -> (38.5013, 17.1827) centre (38.3863, 18.7068) ccw
  arc A441 (38.5013, 17.1827) -> (38.5982, 17.196) centre (38.441, 17.982) ccw
  arc A442 (38.5982, 17.196) -> (38.6694, 17.215) centre (38.483, 17.7717) ccw
  arc A443 (38.6694, 17.215) -> (38.6863, 17.2384) centre (38.6616, 17.2384) ccw
  arc A444 (38.7099, 17.2648) -> (38.6863, 17.2384) centre (38.7128, 17.2384) ccw
  arc A445 (38.8963, 17.2822) -> (38.7099, 17.2648) centre (39.3286, 11.6627) ccw
  arc A446 (39.1418, 17.2946) -> (38.8963, 17.2822) centre (39.2507, 12.6742) ccw
  arc A447 (39.4663, 17.2984) -> (39.1418, 17.2946) centre (39.4663, 3.5337) ccw
  arc A448 (39.8917, 17.2953) -> (39.4663, 17.2984) centre (39.4663, -11.604) ccw
  arc A449 (40.1013, 17.2817) -> (39.8917, 17.2953) centre (39.8608, 15.1977) ccw
  arc A450 (40.2128, 17.2558) -> (40.1013, 17.2817) centre (40.0432, 16.7785) ccw
  arc A451 (40.2463, 17.2084) -> (40.2128, 17.2558) centre (40.196, 17.2084) ccw
  arc A452 (40.2463, 17.2084) -> (40.2677, 17.1646) centre (40.3017, 17.2084) ccw
  arc A453 (40.2677, 17.1646) -> (40.3259, 17.1369) centre (40.3598, 17.2829) ccw
  arc A454 (40.3259, 17.1369) -> (40.4358, 17.1222) centre (40.458, 17.7061) ccw
  arc A455 (40.4358, 17.1222) -> (40.6339, 17.1184) centre (40.6339, 22.3311) ccw
  arc A456 (40.6339, 17.1184) -> (40.9962, 17.1608) centre (40.6339, 18.688) ccw
  arc A457 (40.9962, 17.1608) -> (41.1846, 17.297) centre (40.9262, 17.456) ccw
  arc A458 (41.1846, 17.297) -> (41.2873, 17.5877) centre (40.5601, 17.6811) ccw
  arc A459 (41.2873, 17.5877) -> (41.3627, 18.3034) centre (25.5952, 19.6031) ccw
  line L146 (41.3627, 18.3034) -> (41.4035, 18.7984)
  line L147 (41.4035, 18.7984) -> (40.2176, 18.7984)
  arc A460 (39.5315, 18.8009) -> (40.2176, 18.7984) centre (40.2176, 111.9136) ccw
  arc A461 (39.2444, 18.8136) -> (39.5315, 18.8009) centre (39.5603, 22.7144) ccw
  arc A462 (39.1194, 18.8405) -> (39.2444, 18.8136) centre (39.2838, 19.3004) ccw
  arc A463 (39.1063, 18.8884) -> (39.1194, 18.8405) centre (39.1296, 18.869) ccw
  arc A464 (39.1823, 18.9351) -> (39.1063, 18.8884) centre (39.2131, 18.7998) ccw
  arc A465 (39.3425, 18.9606) -> (39.1823, 18.9351) centre (39.4575, 17.7242) ccw
  arc A466 (39.6042, 18.9748) -> (39.3425, 18.9606) centre (39.6562, 15.5883) ccw
  arc A467 (40.0736, 18.9784) -> (39.6042, 18.9748) centre (40.0736, -11.6067) ccw
  line L148 (40.0736, 18.9784) -> (40.9663, 18.9784)
  line L149 (40.9663, 18.9784) -> (40.9663, 19.6084)
  line L150 (40.9663, 19.6084) -> (40.9663, 20.2384)
  line L151 (40.9663, 20.2384) -> (40.7563, 20.2384)
  arc A468 (40.6758, 20.2427) -> (40.7563, 20.2384) centre (40.7563, 20.9844) ccw
  arc A469 (40.608, 20.256) -> (40.6758, 20.2427) centre (40.7197, 20.647) ccw
  arc A470 (40.5602, 20.2753) -> (40.608, 20.256) centre (40.6758, 20.4933) ccw
  arc A471 (40.5463, 20.2984) -> (40.5602, 20.2753) centre (40.5725, 20.2984) ccw
  arc A472 (40.5667, 20.3232) -> (40.5463, 20.2984) centre (40.5716, 20.2984) ccw
  arc A473 (40.6813, 20.3415) -> (40.5667, 20.3232) centre (40.8927, 18.6504) ccw
  arc A474 (40.8344, 20.3543) -> (40.6813, 20.3415) centre (40.9141, 18.4793) ccw
  arc A475 (41.0263, 20.3584) -> (40.8344, 20.3543) centre (41.0263, 15.838) ccw
  line L152 (41.0263, 20.3584) -> (41.5063, 20.3584)
  line L153 (41.5063, 20.3584) -> (41.5063, 20.5984)
  line L154 (41.5063, 20.5984) -> (41.5063, 20.8384)
  line L155 (41.5063, 20.8384) -> (41.0263, 20.8384)
  arc A476 (40.7382, 20.8415) -> (41.0263, 20.8384) centre (41.0263, 34.2982) ccw
  arc A477 (40.6213, 20.8571) -> (40.7382, 20.8415) centre (40.7495, 21.3701) ccw
  arc A478 (40.5672, 20.8937) -> (40.6213, 20.8571) centre (40.6444, 20.9495) ccw
  arc A479 (40.5463, 20.9584) -> (40.5672, 20.8937) centre (40.6566, 20.9584) ccw
  arc A480 (40.5463, 20.9584) -> (40.5322, 21.0212) centre (40.3989, 20.9584) ccw
  arc A481 (40.5322, 21.0212) -> (40.4938, 21.0574) centre (40.467, 20.9904) ccw
  arc A482 (40.4938, 21.0574) -> (40.4148, 21.0745) centre (40.4036, 20.832) ccw
  arc A483 (40.4148, 21.0745) -> (40.2463, 21.0784) centre (40.2463, 17.4307) ccw
  arc A484 (40.2463, 21.0784) -> (40.0777, 21.0745) centre (40.2463, 17.4307) ccw
  arc A485 (40.0777, 21.0745) -> (39.9988, 21.0574) centre (40.0889, 20.832) ccw
  arc A486 (39.9988, 21.0574) -> (39.9603, 21.0212) centre (40.0256, 20.9904) ccw
  arc A487 (39.9603, 21.0212) -> (39.9463, 20.9584) centre (40.0936, 20.9584) ccw
  arc A488 (39.9276, 20.8942) -> (39.9463, 20.9584) centre (39.8265, 20.9584) ccw
  arc A489 (39.8788, 20.8577) -> (39.9276, 20.8942) centre (39.8552, 20.9401) ccw
  arc A490 (39.7744, 20.8417) -> (39.8788, 20.8577) centre (39.7634, 21.2616) ccw
  arc A491 (39.5263, 20.8384) -> (39.7744, 20.8417) centre (39.5263, 30.2635) ccw
  arc A492 (39.2781, 20.8417) -> (39.5263, 20.8384) centre (39.5263, 30.2635) ccw
  arc A493 (39.1738, 20.8577) -> (39.2781, 20.8417) centre (39.2892, 21.2616) ccw
  arc A494 (39.125, 20.8942) -> (39.1738, 20.8577) centre (39.1973, 20.9401) ccw
  arc A495 (39.1063, 20.9584) -> (39.125, 20.8942) centre (39.2261, 20.9584) ccw
  arc A496 (39.1063, 20.9584) -> (39.0934, 21.0205) centre (38.95, 20.9584) ccw
  arc A497 (39.0934, 21.0205) -> (39.0575, 21.0567) centre (39.029, 20.9926) ccw
  arc A498 (39.0575, 21.0567) -> (38.985, 21.0742) centre (38.9735, 20.8676) ccw